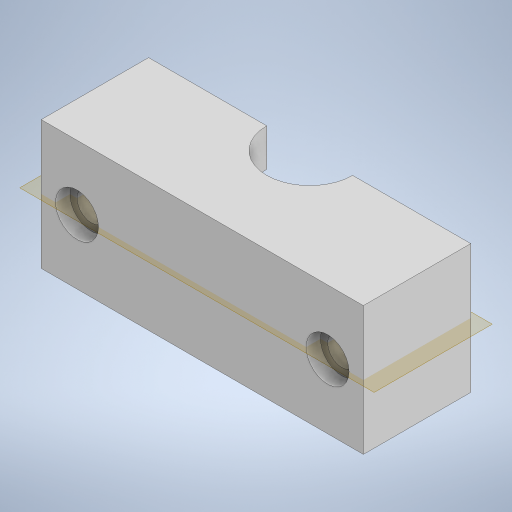
# Autodesk Inventor part: bearing_holder_v2
Saved by Autodesk Inventor 2024 (Build 280153000, 153)
## iProperties
Created: 2024-02-01
Part Number: bearing_holder_v2
Material: Generic
Document SubType Name: Modeling
Designer: Pintu
Density: 1 g/cm^3
Appearance: Default
Author: Pintu
Autodesk Inventor part; units mm, degrees
ref_plane "YZ Plane" through (0, 0, 0) normal (1, 0, 0) x (0, 1, 0)
ref_plane "XZ Plane" through (0, 0, 0) normal (0, 1, 0) x (-1, 0, 0)
ref_plane "XY Plane" through (0, 0, 0) normal (0, 0, 1) x (1, 0, 0)
sketch "Sketch1" plane through (0, 0, 0) normal (0, 0, 1) x (1, 0, 0)
  point P0 (0, 0)
sketch "Sketch2" plane through (0, 0, 0) normal (0, 0, 1) x (1, 0, 0)
  line L0 (-22.5, 9) -> (22.5, 9)
  line L1 (22.5, 9) -> (22.5, -9)
  line L2 (22.5, -9) -> (-22.5, -9)
  line L3 (-22.5, -9) -> (-22.5, 9)
  line L4 (-22.5, 9) -> (22.5, -9) construction
  line L5 (22.5, 9) -> (-22.5, -9) construction
  point P0 (0, 0)
  dimension "d0" = 45
  dimension "d1" = 18
  constraints: 12 end point, 2 midpoint, 2 parallel, 1 horizontal, 1 perpendicular
  measures "d0" distance of L1.end L2.end
  measures "d1" distance of L0.end L1.end
extrude "Extrusion1" add sketch "Sketch2" along normal blind 15
ref_plane "Work Plane1" through (-22.5, 0, 0) normal (0, 1, 0) x (1, 0, 0)
sketch "Sketch3" plane through (-22.5, 0, 0) normal (0, 1, 0) x (1, 0, 0)
  circle A0 centre (22.5, 0) radius 11.5
  dimension "d4" = 23
  constraints: 1 centre point, 1 coincident
  measures "d4" diameter of A0
extrude "Extrusion2" cut sketch "Sketch3" along normal mid plane 7.5
sketch "Sketch4" plane through (-22.5, 0, 0) normal (0, 1, 0) x (1, 0, 0)
  circle A0 centre (22.5, 0) radius 6
  dimension "d7" = 12
  constraints: 1 centre point, 1 coincident
  measures "d7" diameter of A0
extrude "Extrusion3" cut sketch "Sketch4" along normal mid plane 32.75
sketch "Sketch5" plane through (0, 0, 15) normal (0, 0, 1) x (1, 0, 0)
  line L0 (-22.5, 9) -> (-22.5, -9) projected
  line L1 (-22.5, -9) -> (22.5, -9) projected
  point P0 (0, 0)
  point P1 (-17.5, 0)
  dimension "d10" = 5
  dimension "d11" = 9
  measures "d10" distance from line of L0 point (-17.5, 0)
  measures "d11" distance from line of L1 point (-17.5, 0)
hole "Hole1" at (-17.5, 0, 15) direction (0, 0, -1) diameter 4 end through all counterbore diameter 6 counterbore depth 2
sketch "Sketch6" plane through (0, 0, 15) normal (0, 0, 1) x (1, 0, 0)
  line L0 (-22.5, -9) -> (22.5, -9) projected
  line L1 (22.5, -9) -> (22.5, 9) projected
  point P0 (0, 0)
  point P1 (17.5, 0)
  dimension "d19" = 9
  dimension "d20" = 5
  measures "d19" distance from line of L0 point (17.5, 0)
  measures "d20" distance from line of L1 point (17.5, 0)
hole "Hole2" at (17.5, 0, 15) direction (0, 0, -1) diameter 4 end through all counterbore diameter 6 counterbore depth 2
body "Solid1"
